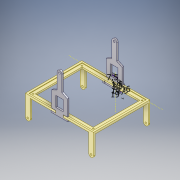
# Autodesk Inventor part: ControllerPCBHolder
Saved by Autodesk Inventor 2019.1 (Build 231200000, 200)
## iProperties
Created: 2018-09-15
Part Number: ControllerPCBHolder
Material: Generisch
Document SubType Name: Modeling
Designer: JochenAlt
Density: 1 g/cm^3
Appearance: Nylon 6
Author: JochenAlt
Autodesk Inventor part; units mm, degrees
ref_plane "YZ Plane" through (0, 0, 0) normal (1, 0, 0) x (0, 1, 0)
ref_plane "XZ Plane" through (0, 0, 0) normal (0, 1, 0) x (-1, 0, 0)
ref_plane "XY Plane" through (0, 0, 0) normal (0, 0, 1) x (1, 0, 0)
sketch "Skizze1" plane through (0, 0, 0) normal (0, 0, 1) x (1, 0, 0)
  line L0 (-61, 50.5) -> (61, 50.5)
  line L1 (61, 50.5) -> (61, -50.5)
  line L2 (61, -50.5) -> (-61, -50.5)
  line L3 (-61, -50.5) -> (-61, 50.5)
  line L4 (0, 70.7) -> (0, -70.7) construction
  line L5 (-85.4, 0) -> (85.4, 0) construction
  line L6 (-55, 44.5) -> (55, 44.5)
  line L7 (55, 44.5) -> (55, -44.5)
  line L8 (55, -44.5) -> (-55, -44.5)
  line L9 (-55, -44.5) -> (-55, 44.5)
  line L10 (-57.15, 46.36) -> (57.15, 46.36) construction
  line L11 (57.15, 46.36) -> (57.15, -46.36) construction
  line L12 (57.15, -46.36) -> (-57.15, -46.36) construction
  line L13 (-57.15, -46.36) -> (-57.15, 46.36) construction
  circle A0 centre (-57.15, 46.36) radius 1.25
  circle A1 centre (57.15, 46.36) radius 1.25
  circle A2 centre (-57.15, -46.36) radius 1.25
  circle A3 centre (57.15, -46.36) radius 1.25
  point P0 (0, 0)
  dimension "d0" = 122
  dimension "d1" = 101
  dimension "d4" = 6
  dimension "d5" = 6
  dimension "d6" = 2.5
  dimension "d7" = 114.3
  dimension "d8" = 92.72
  constraints: 24 end point, 6 parallel, 4 centre point, 4 coincident, 3 equal radius, 3 horizontal, 3 perpendicular, 6 other
  measures "d0" distance of L0.start L0.end
  measures "d1" distance of L0.end L1.end
  measures "d4" distance between parallel lines of L6 L0
  measures "d5" distance between parallel lines of L9 L3
  measures "d6" diameter of A0
  measures "d7" distance of L11.end L12.end
  measures "d8" distance of L10.end L11.end
extrude "Extrusion2" add sketch "Skizze1" along normal blind 3
sketch "Skizze2" plane through (0, 0, 0) normal (0, 1, 0) x (-1, 0, 0)
  arc A0 (55.6888, -34.75) -> (64.6888, -34.75) centre (60.1888, -34.75) ccw
  arc A1 (-64.6888, -34.75) -> (-55.6888, -34.75) centre (-60.1888, -34.75) ccw
  line L0 (0, -98.1) -> (0, 102.1) construction
  line L1 (-97.3, 0) -> (97.3, 0) construction
  circle A2 centre (60.1888, -34.75) radius 1.75
  circle A3 centre (-60.1888, -34.75) radius 1.75
  line L2 (64.6888, -34.75) -> (64.6888, 3)
  line L3 (55.6888, -34.75) -> (55.6888, 3)
  line L4 (-55.6888, -34.75) -> (-55.6888, 3)
  line L5 (-64.6888, -34.75) -> (-64.6888, 3)
  line L6 (-61, 3) -> (61, 3) construction
  line L7 (64.6888, 3) -> (55.6888, 3)
  line L8 (-64.6888, 3) -> (-55.6888, 3)
  circle A4 centre (0, 69.5) radius 1.75
  arc A5 (4.5, 69.5) -> (-4.5, 69.5) centre (0, 69.5) ccw
  line L9 (60.1888, -34.75) -> (0, 69.5) construction
  line L10 (4.5, 69.5) -> (4.5, 39.3)
  line L11 (61, 0) -> (-61, 0) construction
  circle A6 centre (0, 0) radius 69.5 construction
  line L12 (60.1888, -34.75) -> (-60.1888, -34.75) construction
  line L13 (0, 69.5) -> (-60.1888, -34.75) construction
  line L14 (-7.3, 0) -> (-7.3, 4.3)
  line L15 (-7.3, 4.3) -> (-7, 4.3)
  line L16 (7.3, 4.3) -> (7.3, 0)
  line L17 (55, 3) -> (-55, 3) construction
  line L18 (7.3, 0) -> (4.5, 0)
  line L19 (4.5, 0) -> (4.5, 0)
  line L20 (-4.5, 0) -> (-7.3, 0)
  line L21 (4.5, 0) -> (-4.5, 0)
  line L22 (7.3, 4.3) -> (15, 4.3)
  line L23 (15, 4.3) -> (15, 34.3)
  line L24 (15, 34.3) -> (4.5, 39.3)
  line L25 (4.5, 39.3) -> (-4.5, 39.3)
  line L26 (-4.5, 39.3) -> (-15, 34.3)
  line L27 (-15, 34.3) -> (-15, 4.3)
  line L28 (-15, 4.3) -> (-7.3, 4.3)
  line L29 (7, 29.3) -> (-7, 29.3)
  line L30 (7, 29.3) -> (7, 9.3)
  line L31 (-7, 29.3) -> (-4.5, 39.3)
  line L32 (4.5, 39.3) -> (7, 29.3)
  line L33 (-4.5, 39.3) -> (-4.5, 69.5)
  line L34 (7, 9.3) -> (-7, 9.3)
  line L35 (7, 9.3) -> (7, 4.3)
  line L36 (-7, 9.3) -> (-7, 29.3)
  line L37 (-7, 4.3) -> (7.3, 4.3)
  line L38 (-7, 4.3) -> (-7, 9.3)
  line L39 (-7, 4.3) -> (-7, 0)
  line L40 (7, 4.3) -> (7, 0)
  point P0 (0, 0)
  dimension "d12" = 3.5
  dimension "d22" = 69.5
  dimension "d23" = 4.5
  dimension "d44" = 1.3
  dimension "d54" = 30
  dimension "d55" = 5
  dimension "d61" = 30
  dimension "d62" = 14
  dimension "d65" = 0.3
  dimension "d66" = 5
  dimension "d67" = 10
  constraints: 72 end point, 8 point on circle, 8 point on line, 7 centre point, 7 tangent, 7 vertical, 6 horizontal, 6 perpendicular, 5 collinear, 4 coincident, 4 equal radius, 3 equal length, 3 midpoint, 1 parallel, 5 other
  measures "d12" diameter of A2
  measures "d22" radius of A6
  measures "d23" radius of A0
  measures "d44" distance between parallel lines of L17 L15
  measures "d54" distance of L22.end L23.end
  measures "d55" vertical distance of L10.end L23.end
  measures "d61" distance between parallel lines of L27 L23
  measures "d62" distance of L29.start L29.end
  measures "d65" distance between parallel lines of L14 L39
  measures "d66" distance between parallel lines of L37 L34
  measures "d67" distance between parallel lines of L29 L25
extrude "Extrusion3" add sketch "Skizze2" along normal blind 3 from surface at 50.5 contours L3 L7 L2 A0 | L5 L8 L4 A1
extrude "Extrusion4" add sketch "Skizze2" against normal blind 3 from surface at -50.5 contours L3 L7 L2 A0 | L5 L8 L4 A1
sketch "Skizze4" plane through (0, 0, 0) normal (0, 0, 1) x (1, 0, 0)
  line L0 (-64.6888, 53.5) -> (-64.6888, 50.5) projected
  line L1 (55.6888, -53.5) -> (64.6888, -53.5) projected
  line L2 (-64.6888, 53.5) -> (64.6888, 53.5)
  line L3 (64.6888, 53.5) -> (64.6888, -53.5)
  line L4 (64.6888, -53.5) -> (-64.6888, -53.5)
  line L5 (-64.6888, -53.5) -> (-64.6888, 53.5)
  line L6 (61, -50.5) -> (61, 50.5) projected
  line L7 (61, -50.5) -> (-61, -50.5)
  line L8 (-61, -50.5) -> (-61, 50.5)
  line L9 (-61, 50.5) -> (61, 50.5)
  line L10 (61, 50.5) -> (61, -50.5)
  point P0 (0, 0)
  constraints: 16 end point, 4 parallel, 2 horizontal, 2 perpendicular, 1 coincident
extrude "Extrusion5" add sketch "Skizze4" along normal blind 4
extrude "Extrusion7" cut sketch "Skizze2" along normal up to surface (3 mm away) from surface at -53.5 contours L40 L18 L21 L20 L39 L37
extrude "Extrusion8" cut sketch "Skizze2" against normal up to surface (3 mm away) from surface at 53.5 contours L40 L18 L21 L20 L39 L37
sketch "Skizze5" plane through (0, 0, 0) normal (0, 1, 0) x (-1, 0, 0)
  point P0 (0, 0)
sketch "Skizze6" plane through (-55.6888, 53.5, 0) normal (0, -1, 0) x (1, 0, 0)
  line L0 (-34.8755, 0) -> (146.253, 0) construction
  line L1 (55.6888, 19.25) -> (55.6888, -49) construction
  line L2 (44.6888, 7.5) -> (63.6888, 7.5)
  line L3 (63.6888, 7.5) -> (63.6888, -8.5)
  line L4 (63.6888, -8.5) -> (44.6888, -8.5)
  line L5 (44.6888, -8.5) -> (44.6888, 7.5)
  line L6 (111.3775, 0) -> (0, 0) projected
  circle A0 centre (47.1888, -6) radius 1.75
  circle A1 centre (61.1888, -6) radius 1.75
  line L7 (61.1888, -6) -> (47.1888, -6) construction
  line L8 (54.1888, 7.5) -> (54.1888, -8.5) construction
  line L9 (42.6888, -10.5) -> (65.6888, -10.5)
  line L10 (65.6888, -10.5) -> (65.6888, 9.5)
  line L11 (65.6888, 9.5) -> (42.6888, 9.5)
  line L12 (42.6888, 9.5) -> (42.6888, -10.5)
  circle A2 centre (61.1888, -6) radius 3.25
  circle A3 centre (47.1888, -6) radius 3.25
  point P0 (55.6888, 0)
  point P1 (55.6888, 0)
  point P2 (55.6888, 0)
  dimension "d24" = 19
  dimension "d25" = 16
  dimension "d29" = 7.5
  dimension "d30" = 3.5
  dimension "d31" = 2.5
  dimension "d32" = 14
  dimension "d33" = 8
  dimension "d48" = 2
  dimension "d58" = 1.5
  constraints: 20 end point, 4 centre point, 4 parallel, 3 coincident, 3 midpoint, 3 perpendicular, 2 equal radius, 2 horizontal, 1 symmetric about line, 4 other
  measures "d24" distance of L3.end L4.end
  measures "d25" distance of L2.end L3.end
  measures "d29" distance from line of L2 point (55.689, 0)
  measures "d30" diameter of A0
  measures "d31" distance from line of L4 L7.start
  measures "d32" distance of L7.start L7.end
  measures "d33" distance between parallel lines of L3 L1
  measures "d48" distance between parallel lines of L4 L9
  measures "d58" radial gap between concentric circles of A2 A1
extrude "Extrusion6" add sketch "Skizze2" against normal up to surface (3 mm away) from surface at -50.5 separate body contours L10 L25 L33 A5 | L32 L29 L31 L25 | L24 L23 L22 L37 L35 L30 L32 | L31 L36 L38 L15 L28 L27 L26 | L35 L37 L38 L34 | L16 L18 L40 L37 | L40 L18 L21 L20 L39 L37 | L15 L39 L20 L14
extrude "Extrusion9" add sketch "Skizze2" against normal up to surface (3 mm away) from surface at 53.5 contours L10 L25 L33 A5 | L32 L29 L31 L25 | L24 L23 L22 L37 L35 L30 L32 | L31 L36 L38 L15 L28 L27 L26 | L35 L37 L38 L34 | L16 L18 L40 L37 | L40 L18 L21 L20 L39 L37 | L15 L39 L20 L14 bodies 2
sketch "Skizze7" plane through (4, -53.5, 0) normal (0, 0, -1) x (-1, 0, 0)
  line L0 (-51.6888, 0) -> (59.6888, 0) construction
  line L1 (20, 0) -> (20, 0)
  line L2 (-12, 0) -> (-12, 9)
  line L3 (-12, 9) -> (20, 9)
  line L4 (20, 9) -> (20, 0)
  line L5 (59, 9) -> (-51, 9) construction
  line L6 (20, 107) -> (-12, 107)
  line L7 (-12, 107) -> (-12, 98)
  line L8 (-12, 98) -> (20, 98)
  line L9 (20, 98) -> (20, 107)
  line L10 (59, 98) -> (-51, 98) projected
  line L11 (-60.6888, 107) -> (68.6888, 107) projected
  line L12 (8.5, 3) -> (8.5, 0) construction
  line L13 (-0.5, 3) -> (-0.5, 0) construction
  line L14 (2.25, 3) -> (5.75, 3) construction
  line L15 (2.25, 0) -> (5.75, 0) construction
  line L16 (11, 3) -> (-0.5, 3) construction
  line L17 (4, 3) -> (4, 0) construction
  line L18 (8.5, 0) -> (-0.5, 0) construction
  line L19 (20, 9) -> (20, 0)
  line L20 (20, 9) -> (20, 9)
  line L21 (20, 0) -> (-12, 0)
  point P0 (4, 53.5)
  point P1 (8.65, 0)
  point P2 (-0.15, 107)
  point P3 (8.65, 3)
  dimension "d45" = 32
  dimension "d51" = 16
  constraints: 24 end point, 7 parallel, 5 point on line, 3 horizontal, 3 perpendicular, 2 collinear, 1 midpoint, 1 other
  measures "d45" distance between parallel lines of L2 L4
  measures "d51" distance between parallel lines of L17 L2
extrude "Extrusion10" add sketch "Skizze7" along normal blind 3 contours L9 L8 L7 L6 bodies 2
extrude "Extrusion12" add sketch "Skizze7" along normal blind 3 contours L2 L3 L4 L21 bodies 2
extrude "Extrusion11" add sketch "Skizze6" against normal blind 4 bodies 2
extrude "Extrusion13" add sketch "Skizze6" against normal blind 5 from surface at -4 contours A3 L4 L5 | L5 A3 | A2 L3 | L3 A2 L4 | L4 A2 | L4 A3 picked at (47.2591, -8.2457) picked at (61.1185, -8.2457) bodies 2
equation "\"d5\" = d4"
